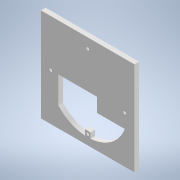
# Autodesk Inventor part: Base
Saved by Autodesk Inventor 2020 (Build 240168000, 168)
## iProperties
Created: 2020-08-08
Part Number: Base
Material: Generic
Document SubType Name: Modeling
Designer: reide
Density: 1 g/cm^3
Appearance: Default
Author: reide
Autodesk Inventor part; units mm, degrees
ref_plane "YZ Plane" through (0, 0, 0) normal (1, 0, 0) x (0, 1, 0)
ref_plane "XZ Plane" through (0, 0, 0) normal (0, 1, 0) x (-1, 0, 0)
ref_plane "XY Plane" through (0, 0, 0) normal (0, 0, 1) x (1, 0, 0)
sketch "Sketch1" plane through (0, 0, 0) normal (0, 0, 1) x (1, 0, 0)
  line L0 (-50, 50) -> (50, 50)
  line L1 (50, 50) -> (50, -50)
  line L2 (50, -50) -> (-50, -50)
  line L3 (-50, -50) -> (-50, 50)
  line L4 (-50, 50) -> (50, -50) construction
  line L5 (50, 50) -> (-50, -50) construction
  arc A0 (3, -42.394) -> (42.394, -3) centre (0, 0) ccw projected
  arc A1 (42.394, 3) -> (3, 42.394) centre (0, 0) ccw projected
  circle A2 centre (39.5, 0) radius 1.25 projected
  circle A3 centre (0, -39.5) radius 1.25 projected
  circle A4 centre (0, 39.5) radius 1.25 projected
  circle A5 centre (-39.5, 0) radius 1.25 projected
  circle A6 centre (0, 0) radius 47.5 projected
  arc A7 (3, -42.394) -> (42.394, -3) centre (0, 0) ccw projected
  line L6 (3, -42.394) -> (3, -36.5) projected
  line L7 (3, -36.5) -> (-3, -36.5) projected
  line L8 (-3, -36.5) -> (-3, -42.394) projected
  arc A8 (-42.394, -3) -> (-3, -42.394) centre (0, 0) ccw projected
  line L9 (-42.394, -3) -> (-36.5, -3) projected
  line L10 (-36.5, -3) -> (-36.5, 3) projected
  line L11 (-36.5, 3) -> (-42.394, 3) projected
  arc A9 (-3, 42.394) -> (-42.394, 3) centre (0, 0) ccw projected
  line L12 (-3, 42.394) -> (-3, 36.5) projected
  line L13 (-3, 36.5) -> (3, 36.5) projected
  line L14 (3, 36.5) -> (3, 42.394) projected
  arc A10 (42.394, 3) -> (3, 42.394) centre (0, 0) ccw projected
  line L15 (42.394, 3) -> (36.5, 3) projected
  line L16 (36.5, 3) -> (36.5, -3) projected
  line L17 (36.5, -3) -> (42.394, -3) projected
  circle A11 centre (0, 0) radius 42.5
  circle A12 centre (39.5, 0) radius 1.5
  circle A13 centre (0, -39.5) radius 1.5
  circle A14 centre (0, 39.5) radius 1.5
  circle A15 centre (-39.5, 0) radius 1.5
  line L18 (36.5, 0) -> (-36.5, 0)
  line L19 (0, 0) -> (10, 0)
  line L20 (10, 0) -> (10, -15)
  line L21 (10, -15) -> (39.7649, -15)
  line L22 (-36.5, 0) -> (-31.5, 0)
  line L23 (-31.5, 0) -> (-31.5, -28.5307)
  point P0 (0, 0)
  dimension "d0" = 100
  dimension "d1" = 100
  dimension "d2" = 3
  dimension "d3" = 3
  dimension "d4" = 3
  dimension "d5" = 3
  dimension "d8" = 10
  dimension "d9" = 15
  dimension "d10" = 5
  constraints: 24 end point, 5 centre point, 5 coincident, 4 midpoint, 3 perpendicular, 2 parallel, 2 point on circle, 2 point on line, 1 concentric, 1 horizontal, 1 vertical
  measures "d0" distance of L0.start L0.end
  measures "d1" distance of L0.end L1.end
  measures "d2" diameter of A12
  measures "d3" diameter of A13
  measures "d4" diameter of A14
  measures "d5" diameter of A15
  measures "d8" distance of L19.start L19.end
  measures "d9" distance of L19.end L20.end
  measures "d10" distance of L18.end L22.end
extrude "Extrusion1" add sketch "Sketch1" along normal blind 5 contours L0 L1 L2 L3 | A11 L8 L7 L6 | L21 L20 L18 L16 L17 A0 | L17 L16 L15 A11 | A8 L9 L10 L18 L23 | L18 L10 L11 A9 L12 L13 L14 A1 L15 L16 | A11 L11 L10 L9 | L14 L13 L12 A11 | A6
sketch "Sketch2" plane through (0, 0, 5) normal (0, 0, 1) x (1, 0, 0)
  circle A0 centre (14, 43) radius 1.4 projected
  circle A1 centre (14, -6) radius 1.4 projected
  circle A2 centre (-44, 43) radius 1.4 projected
  circle A3 centre (-44, -6) radius 1.4 projected
  circle A4 centre (-44, 43) radius 3.5
  circle A5 centre (-44, -6) radius 3.5
  circle A6 centre (14, 43) radius 3.5
  circle A7 centre (14, -6) radius 3.5
  circle A8 centre (14, -6) radius 1.4
  circle A9 centre (14, 43) radius 1.4
  circle A10 centre (14, 43) radius 1.3
  circle A11 centre (14, -6) radius 1.3
  circle A12 centre (-44, 43) radius 1.3
  circle A13 centre (-44, -6) radius 1.3
  point P0 (0, 0)
  dimension "d11" = 7
  dimension "d12" = 7
  dimension "d13" = 7
  dimension "d14" = 7
  dimension "d15" = 2.6
  dimension "d16" = 2.6
  dimension "d17" = 2.6
  dimension "d18" = 2.6
  constraints: 10 centre point, 10 coincident, 2 concentric
  measures "d11" diameter of A4
  measures "d12" diameter of A5
  measures "d13" diameter of A6
  measures "d14" diameter of A7
  measures "d15" diameter of A10
  measures "d16" diameter of A11
  measures "d17" diameter of A12
  measures "d18" diameter of A13
extrude "Extrusion2" add sketch "Sketch2" along normal blind 5 contours A0 | A1 | A2 | A3 | A4 | A5 | A6 | A7
fillet "Fillet1" radius 2 5 edges at (10, -15, 2.5) (39.7649, -15, 2.5) (-31.5, 0, 2.5) (10, 0, 2.5) (-31.5, -28.5307, 2.5)
sketch "Sketch3" plane through (0, 0, 5) normal (0, 0, 1) x (1, 0, 0)
  circle A0 centre (0, 0) radius 47.5 projected
  circle A1 centre (0, -39.5) radius 1.5 projected
  circle A2 centre (39.5, 0) radius 1.5 projected
  circle A3 centre (0, 39.5) radius 1.5 projected
  circle A4 centre (-39.5, 0) radius 1.5 projected
  arc A5 (10, -13) -> (12, -15) centre (12, -13) ccw projected
  line L0 (12, -15) -> (36.7594, -15) projected
  arc A6 (38.5746, -17.8395) -> (36.7594, -15) centre (36.7594, -17) ccw projected
  arc A7 (3, -42.394) -> (38.5746, -17.8395) centre (0, 0) ccw projected
  line L1 (3, -42.394) -> (3, -36.5) projected
  line L2 (3, -36.5) -> (-3, -36.5) projected
  line L3 (-3, -36.5) -> (-3, -42.394) projected
  arc A8 (-30.9568, -29.1192) -> (-3, -42.394) centre (0, 0) ccw projected
  arc A9 (-31.5, -27.7489) -> (-30.9568, -29.1192) centre (-29.5, -27.7489) ccw projected
  line L4 (-31.5, -27.7489) -> (-31.5, -2) projected
  arc A10 (-29.5, 0) -> (-31.5, -2) centre (-29.5, -2) ccw projected
  line L5 (-29.5, 0) -> (8, 0) projected
  arc A11 (10, -2) -> (8, 0) centre (8, -2) ccw projected
  line L6 (10, -2) -> (10, -13) projected
  line L7 (-50, 50) -> (-50, -50) projected
  line L8 (-50, -50) -> (50, -50) projected
  line L9 (50, -50) -> (50, 50) projected
  line L10 (50, 50) -> (-50, 50) projected
  circle A12 centre (14, 43) radius 3.5 projected
  circle A13 centre (-44, -6) radius 3.5 projected
  circle A14 centre (14, -6) radius 3.5 projected
  circle A15 centre (-44, 43) radius 3.5 projected
  line L11 (14.5, 46.5) -> (-44.5, 46.5) projected
  line L12 (48, 48) -> (-48, 48)
  line L13 (-48, 48) -> (-48, -48)
  line L14 (-48, -48) -> (48, -48)
  line L15 (48, -48) -> (48, 48)
  line L16 (48, 48) -> (-48, -48) construction
  line L17 (-48, 48) -> (48, -48) construction
  line L18 (-50, 50) -> (-50, -50) projected
  point P0 (0, 0)
  dimension "d22" = 96
  dimension "d23" = 96
  constraints: 12 end point, 2 midpoint, 2 parallel, 2 perpendicular
  measures "d22" distance of L12.start L12.end
  measures "d23" distance of L13.end L12.end
extrude "Extrusion3" add sketch "Sketch3" along normal blind 30 contours L10 L9 L8 L7
sketch "Sketch4" plane through (-50, -50, 0) normal (-1, 0, 0) x (0, 0, 1)
  line L0 (12.6725, 57.7) -> (19.7725, 57.7) projected
  line L1 (19.7725, 72.4) -> (19.7725, 57.7) projected
  line L2 (12.6725, 72.4) -> (19.7725, 72.4) projected
  line L3 (12.6725, 57.7) -> (12.6725, 72.4) projected
  line L4 (11.9725, 73.05) -> (11.9725, 57.05)
  line L5 (11.9725, 57.05) -> (20.4725, 57.05)
  line L6 (20.4725, 57.05) -> (20.4725, 73.05)
  line L7 (20.4725, 73.05) -> (11.9725, 73.05)
  line L8 (11.9725, 73.05) -> (20.4725, 57.05) construction
  line L9 (11.9725, 57.05) -> (20.4725, 73.05) construction
  point P0 (0, 50)
  point P1 (16.2225, 65.05)
  dimension "d26" = 16
  dimension "d27" = 8.5
  constraints: 12 end point, 2 midpoint, 2 parallel, 1 perpendicular, 1 vertical
  measures "d26" distance of L4.start L4.end
  measures "d27" distance of L5.end L4.end
extrude "Extrusion4" cut sketch "Sketch4" against normal blind 30 contours L3 L2 L1 L0 | L7 L6 L5 L4
fillet "Fillet2" radius 0.5 4 edges at (-49, 23.05, 20.4725) (-49, 7.05, 20.4725) (-49, 7.05, 11.9725) (-49, 23.05, 11.9725)
fillet "Fillet3" radius 0.5 8 edges at (-50, 7.1964, 20.326) (-50, 7.05, 16.2225) (-50, 7.1964, 12.1189) (-50, 15.05, 11.9725) (-50, 22.9036, 12.1189) (-50, 23.05, 16.2225) (-50, 22.9036, 20.326) (-50, 15.05, 20.4725)
fillet "Fillet4" radius 0.5 8 edges at (-48, 22.9036, 12.1189) (-48, 15.05, 11.9725) (-48, 7.1964, 12.1189) (-48, 7.05, 16.2225) (-48, 7.1964, 20.326) (-48, 15.05, 20.4725) (-48, 22.9036, 20.326) (-48, 23.05, 16.2225)
sketch "Sketch5" plane through (-50, 50, 0) normal (0, 1, 0) x (1, 0, 0)
  circle A0 centre (14, -15.6725) radius 1.875 projected
  circle A1 centre (14, -15.6725) radius 2.25
  point P0 (50, 0)
  dimension "d33" = 4.5
  constraints: 1 centre point, 1 coincident
  measures "d33" diameter of A1
extrude "Extrusion5" cut sketch "Sketch5" against normal blind 30 contours A0 | A1
sketch "Sketch6" plane through (-50, 50, 0) normal (0, 1, 0) x (1, 0, 0)
  line L0 (42.75, -19.1725) -> (28.25, -19.1725) projected
  line L1 (42.75, -12.6725) -> (28.25, -12.6725) projected
  line L2 (28.25, -12.6725) -> (28.25, -19.1725) projected
  line L3 (42.75, -19.1725) -> (28.25, -19.1725) projected
  line L4 (42.75, -12.6725) -> (42.75, -19.1725) projected
  arc A0 (28.5, -18.3475) -> (29, -18.8475) centre (29, -18.3475) ccw projected
  line L5 (28.5, -18.3475) -> (28.5, -16.2524) projected
  arc A1 (28.7925, -15.7975) -> (28.5, -16.2524) centre (29, -16.2524) ccw projected
  arc A2 (28.7925, -15.7975) -> (29.8148, -15.2136) centre (28.0748, -13.3538) ccw projected
  line L6 (29.8148, -15.2136) -> (30.3999, -14.4845) projected
  arc A3 (30.7898, -14.2975) -> (30.3999, -14.4845) centre (30.7898, -14.7975) ccw projected
  line L7 (30.7898, -14.2975) -> (40.2102, -14.2975) projected
  arc A4 (40.6001, -14.4845) -> (40.2102, -14.2975) centre (40.2102, -14.7975) ccw projected
  line L8 (40.6001, -14.4845) -> (41.1852, -15.2136) projected
  arc A5 (41.1852, -15.2136) -> (41.55, -15.4975) centre (41.9651, -14.5877) ccw projected
  line L9 (41.55, -15.4975) -> (42.2075, -15.7975) projected
  arc A6 (42.5, -16.2524) -> (42.2075, -15.7975) centre (42, -16.2524) ccw projected
  line L10 (42.5, -16.2524) -> (42.5, -18.3475) projected
  arc A7 (42, -18.8475) -> (42.5, -18.3475) centre (42, -18.3475) ccw projected
  line L11 (42, -18.8475) -> (29, -18.8475) projected
  line L12 (60.92, -12.6725) -> (52.88, -12.6725) projected
  line L13 (52.88, -12.6725) -> (52.88, -15.6725) projected
  line L14 (60.92, -15.6725) -> (52.88, -15.6725) projected
  line L15 (60.92, -12.6725) -> (60.92, -15.6725) projected
  line L16 (53.5746, -14.4698) -> (54.2077, -13.8575) projected
  line L17 (54.2077, -13.8575) -> (59.3923, -13.8575) projected
  line L18 (59.3923, -13.8575) -> (60.0254, -14.4698) projected
  arc A8 (60.04, -14.5052) -> (60.0254, -14.4698) centre (59.99, -14.5052) ccw projected
  line L19 (60.04, -14.5052) -> (60.04, -15.2375) projected
  arc A9 (59.99, -15.2875) -> (60.04, -15.2375) centre (59.99, -15.2375) ccw projected
  line L20 (59.99, -15.2875) -> (53.61, -15.2875) projected
  arc A10 (53.56, -15.2375) -> (53.61, -15.2875) centre (53.61, -15.2375) ccw projected
  line L21 (53.56, -15.2375) -> (53.56, -14.5052) projected
  arc A11 (53.5746, -14.4698) -> (53.56, -14.5052) centre (53.61, -14.5052) ccw projected
  line L22 (47, -9.482) -> (24, -9.482)
  line L23 (24, -9.482) -> (24, -22.482)
  line L24 (24, -22.482) -> (47, -22.482)
  line L25 (47, -22.482) -> (47, -9.482)
  line L26 (47, -9.482) -> (24, -22.482) construction
  line L27 (24, -9.482) -> (47, -22.482) construction
  line L28 (62.8, -10.1636) -> (50.8, -10.1636)
  line L29 (50.8, -10.1636) -> (50.8, -18.1636)
  line L30 (50.8, -18.1636) -> (62.8, -18.1636)
  line L31 (62.8, -18.1636) -> (62.8, -10.1636)
  line L32 (62.8, -10.1636) -> (50.8, -18.1636) construction
  line L33 (50.8, -10.1636) -> (62.8, -18.1636) construction
  point P0 (50, 0)
  point P1 (35.5, -15.982)
  point P2 (56.8, -14.1636)
  dimension "d36" = 23
  dimension "d37" = 13
  dimension "d40" = 12
  dimension "d41" = 8
  constraints: 24 end point, 4 midpoint, 4 parallel, 4 perpendicular
  measures "d36" distance of L22.start L22.end
  measures "d37" distance of L23.end L22.end
  measures "d40" distance of L28.start L28.end
  measures "d41" distance of L29.end L28.end
extrude "Extrusion6" cut sketch "Sketch6" against normal blind 30 contours L0 L2 L1 L4 | L5 A1 A2 L6 A3 L7 A4 L8 A5 L9 A6 L10 A7 L11 A0 | L15 L14 L13 L12 | L16 L17 L18 A8 L19 A9 L20 A10 L21 A11 | L25 L24 L23 L22 | L31 L30 L29 L28
fillet "Fillet5" radius 0.5 8 edges at (12.8, 49, 18.1636) (12.8, 49, 10.1636) (0.8, 49, 18.1636) (0.8, 49, 10.1636) (-26, 49, 9.482) (-3, 49, 9.482) (-26, 49, 22.482) (-3, 49, 22.482)
fillet "Fillet6" radius 0.5 32 edges at (0.9464, 50, 18.0172) (0.8, 50, 14.1636) (0.9464, 50, 10.3101) (6.8, 50, 10.1636) (12.6536, 50, 10.3101) (12.8, 50, 14.1636) (12.6536, 50, 18.0172) (6.8, 50, 18.1636) (12.6536, 48, 18.0172) (12.8, 48, 14.1636) (12.6536, 48, 10.3101) (6.8, 48, 10.1636) (0.9464, 48, 10.3101) (0.8, 48, 14.1636) (0.9464, 48, 18.0172) (6.8, 48, 18.1636) (-3.1464, 48, 22.3355) (-3, 48, 15.982) (-3.1464, 48, 9.6284) (-14.5, 48, 9.482) (-25.8536, 48, 9.6284) (-26, 48, 15.982) (-25.8536, 48, 22.3355) (-14.5, 48, 22.482) (-3.1464, 50, 22.3355) (-14.5, 50, 22.482) (-25.8536, 50, 22.3355) (-26, 50, 15.982) (-25.8536, 50, 9.6284) (-14.5, 50, 9.482) (-3.1464, 50, 9.6284) (-3, 50, 15.982)
fillet "Fillet7" radius 0.5 2 edges at (-38.25, 48, 15.6725) (-38.25, 50, 15.6725)
fillet "Fillet8" radius 3 4 edges at (-50, 50, 17.5) (50, 50, 17.5) (-50, -50, 17.5) (50, -50, 17.5)
fillet "Fillet9" radius 3 8 edges at (49.1213, 49.1213, 0) (0, 50, 0) (-49.1213, 49.1213, 0) (-50, 0, 0) (-49.1213, -49.1213, 0) (0, -50, 0) (49.1213, -49.1213, 0) (50, 0, 0)
sketch "Sketch7" plane through (0, 0, 35) normal (0, 0, 1) x (1, 0, 0)
  line L0 (48, -48) -> (48, 48) projected
  line L1 (48, 0) -> (48, -3)
  line L2 (48, -3) -> (48, 3)
  line L3 (48, 3) -> (42, 3)
  line L4 (42, 3) -> (48, 3)
  line L5 (48, 3) -> (48, -3)
  line L6 (48, -3) -> (42, -3)
  line L7 (42, -3) -> (42, 3)
  circle A0 centre (45, 0) radius 1.25
  line L8 (0, 48) -> (3, 48)
  line L9 (3, 48) -> (-3, 48)
  line L10 (-3, 48) -> (-3, 42)
  line L11 (-3, 42) -> (-3, 48)
  line L12 (-3, 48) -> (3, 48)
  line L13 (3, 48) -> (3, 42)
  line L14 (3, 42) -> (-3, 42)
  circle A1 centre (0, 45) radius 1.25
  line L15 (-48, 0) -> (-48, 3)
  line L16 (-48, 3) -> (-48, -3)
  line L17 (-48, -3) -> (-42, -3)
  line L18 (-42, -3) -> (-48, -3)
  line L19 (-48, -3) -> (-48, 3)
  line L20 (-48, 3) -> (-42, 3)
  line L21 (-42, 3) -> (-42, -3)
  circle A2 centre (-45, 0) radius 1.25
  line L22 (0, -48) -> (-3, -48)
  line L23 (-3, -48) -> (3, -48)
  line L24 (3, -48) -> (3, -42)
  line L25 (3, -42) -> (3, -48)
  line L26 (3, -48) -> (-3, -48)
  line L27 (-3, -48) -> (-3, -42)
  line L28 (-3, -42) -> (3, -42)
  circle A3 centre (0, -45) radius 1.25
  point P0 (0, 0)
  dimension "d47" = 3
  dimension "d48" = 6
  dimension "d49" = 6
  dimension "d50" = 2.5
  dimension "d53" = 360
  constraints: 56 end point, 4 centre point, 2 parallel, 2 perpendicular, 2 point on line, 1 horizontal, 1 midpoint, 61 other
  measures "d47" distance of L1.start L1.end
  measures "d48" distance of L1.end L2.end
  measures "d49" distance of L2.end L3.end
  measures "d50" diameter of A0
extrude "Extrusion7" add sketch "Sketch7" against normal blind 5
fillet "Fillet10" radius 1 16 edges at (42, -3, 32.5) (3, 42, 32.5) (-3, 42, 32.5) (-3, 48, 32.5) (48, -3, 32.5) (42, 3, 32.5) (48, 3, 32.5) (3, -42, 32.5) (-3, -42, 32.5) (-3, -48, 32.5) (3, -48, 32.5) (3, 48, 32.5) (-48, 3, 32.5) (-42, 3, 32.5) (-42, -3, 32.5) (-48, -3, 32.5)
fillet "Fillet11" radius 1 16 edges at (24.3797, -15, 5) (10.5858, -14.4142, 5) (10, -7.5, 5) (-10.75, 0, 5) (-31.5, -14.8744, 5) (-31.3592, -28.4859, 5) (-18.2297, -38.3918, 5) (24.1421, -34.9772, 5) (24.3797, -15, 0) (10.5858, -14.4142, 0) (10, -7.5, 0) (-10.75, 0, 0) (-31.5, -14.8744, 0) (-31.3592, -28.4859, 0) (-18.2297, -38.3918, 0) (24.1421, -34.9772, 0)
fillet "Fillet12" radius 1 4 edges at (3, -36.5, 2.5) (-3, -36.5, 2.5) (3, -42.394, 2.5) (-3, -42.394, 2.5)
body "Solid1"
